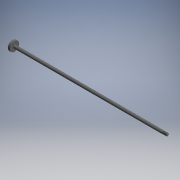
# Autodesk Inventor part: CE263-800_ROD
Saved by Autodesk Inventor 2017.3 (Build 213256000, 256)
## iProperties
Part Number: CE263-800_ROD
Material: Generic
Catalog Web Link: www.cadenas.de
Description: CE2 ROD-Stroke Reading Cylinder with Brake
Vendor: SMC
Document SubType Name: Modeling
Designer: partserver
Manufacturer: SMC
Mass: 372.792 g
Surface Area: 745.586 cm^2
Volume: 372.792 cm^3
Density: 1 g/cm^3
Appearance: PSOLRGB-128-128-128
Category: PARTsolutions
Company: SMC
Title: CE263-800_ROD
Author: Cadenas PARTsolutions
Comments: Stroke Reading Cylinder with Brake
PSOL_IDENT_0: {$CADENAS_DATA\23d-libs\smc_jp\actuator\stroke_reading_cylinders\ce2\parts\ce2_rod.prj},188 {VTYP=3D
PSOL_IDENT_1: },{NB=CE263-800_ROD},{LINA=CE263-800_ROD},{NN=CE2 ROD},{DATE=05.07.2021 01:49:17},{GEOMDATE=15.05.20
PSOL_IDENT_2: 19 00:10:08},{VERSION=},{LINEID=150},{WBVAR=SUFFIX1,STROKE},{WBNUMERIC=STROKE}  {NB=CE263-800_ROD},{
PSOL_IDENT_3: LINA=CE263-800_ROD},{KT=DUMMY},{ORDER=CE263-800},{BORE=63},{SUFFIX1=},{STROKE=800},{A=35.000},{AL=32
PSOL_IDENT_4: .000},{BL=27.000},{D=20.000},{H1=11.000},{K=9.000},{MM=M18x1.5},{NN=187.000},{H=58.000},{HH=66.000},
PSOL_IDENT_5: {LX=200},{MMRA=18.000}
NB: CE263-800_ROD
NN: 187
NT: Stroke Reading Cylinder with Brake
NBSYN: $ORDER._ROD
LINA: CE263-800_ROD
CATALOG: SMC (JP
BORE: 63
SUFFIX1: (-) Without rod boot
STROKE: 800
A: 35
AL: 32
BL: 27
D: 20
H1: 11
K: 9
MM: M18x1.5
H: 58
HH: 66
MMRA: 18
SUPPLIER: SMC
ARTICLENO: CE263-800_ROD
BOMINFO: CE263-800_ROD
CREATOR: CADENAS GmbH
Autodesk Inventor part; units mm, degrees
sketch "Sketch_1" plane through (0, 0, 0) normal (0, 0, 1) x (1, 0, 0)
  line L0 (1002, 0) -> (-58, 0)
  line L1 (-58, 0) -> (-58, 8.08)
  line L2 (-58, 8.08) -> (-57.08, 9)
  line L3 (-57.08, 9) -> (-23, 9)
  line L4 (-23, 9) -> (-21.2679, 10)
  line L5 (-21.2679, 10) -> (987, 10)
  line L6 (987, 10) -> (987, 31.5)
  line L7 (987, 31.5) -> (1002, 31.5)
  line L8 (1002, 31.5) -> (1002, 0)
  line L9 (1002, 0) -> (-58, 0)
  constraints: 20 end point
revolve "Revolution1" add sketch "Sketch_1" angle 360 about axis through (1002, 0, 0) along (1, 0, 0)
thread "Thread1" size "M18x1.5" class "6g" standard "ISO Metric profile" length 31.08
sketch "Sketch_2" plane through (0, 0, 0) normal (0, 1, 0) x (-1, 0, 0)
  line L0 (23, -10) -> (23, -9)
  line L1 (23, -9) -> (14, -9)
  line L2 (14, -9) -> (13, -10)
  line L3 (13, -10) -> (23, -10)
  constraints: 8 end point
extrude "Extrusion1" cut sketch "Sketch_2" along normal mid plane 20
sketch "Sketch_3" plane through (0, 0, 0) normal (0, 1, 0) x (-1, 0, 0)
  line L0 (23, 10) -> (13, 10)
  line L1 (13, 10) -> (14, 9)
  line L2 (14, 9) -> (23, 9)
  line L3 (23, 9) -> (23, 10)
  constraints: 8 end point
extrude "Extrusion2" cut sketch "Sketch_3" along normal mid plane 20
ref_plane "K_XY" through (-14, 0, 0) normal (0, 0, 1) x (1, 0, 0)
ref_plane "K_YZ" through (-14, 0, 0) normal (1, 0, 0) x (0, 1, 0)
ref_plane "K_ZX" through (-14, 0, 0) normal (0, 1, 0) x (0, 0, 1)
ref_plane "rod_XY" through (0, 0, 0) normal (1, 0, 0) x (0, 0, -1)
ref_plane "rod_YZ" through (0, 0, 0) normal (0, 0, -1) x (0, 1, 0)
ref_plane "rod_ZX" through (0, 0, 0) normal (0, 1, 0) x (1, 0, 0)
ref_plane "rod_nut_XY" through (-42, 0, 0) normal (-1, 0, 0) x (0, 0, -1)
ref_plane "rod_nut_YZ" through (-42, 0, 0) normal (0, 0, -1) x (0, -1, 0)
ref_plane "rod_nut_ZX" through (-42, 0, 0) normal (0, -1, 0) x (-1, 0, 0)
body "Solid1"
